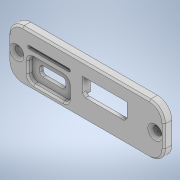
# Autodesk Inventor part: cover
Saved by Autodesk Inventor 2021 (Build 250183000, 183)
## iProperties
Created: 2025-12-12
Part Number: cover
Material: Generic
Document SubType Name: Modeling
Designer: Toby
Density: 1 g/cm^3
Appearance: Default
Author: Toby
Autodesk Inventor part; units mm, degrees
ref_plane "YZ Plane" through (0, 0, 0) normal (1, 0, 0) x (0, 1, 0)
ref_plane "XZ Plane" through (0, 0, 0) normal (0, 1, 0) x (-1, 0, 0)
ref_plane "XY Plane" through (0, 0, 0) normal (0, 0, 1) x (1, 0, 0)
sketch "Sketch1" plane through (0, 0, 0) normal (0, 0, 1) x (1, 0, 0)
  line L0 (-27, 8.75) -> (27, 8.75)
  line L1 (27, 8.75) -> (27, -8.75)
  line L2 (27, -8.75) -> (-27, -8.75)
  line L3 (-27, -8.75) -> (-27, 8.75)
  point P0 (0, 0)
  dimension "d0" = 17.5
  dimension "d1" = 54
  dimension "d2" = 8.75
  dimension "d3" = 27
  constraints: 8 end point, 2 parallel, 1 horizontal, 1 perpendicular
  measures "d0" distance of L2.end L0.start
  measures "d1" distance of L0.start L0.end
  measures "d2" distance from line of point (0, 0) L0
  measures "d3" distance from line of point (0, 0) L3
extrude "Extrusion1" add sketch "Sketch1" along normal blind 2.8
fillet "Fillet1" radius 5 4 edges at (-27, 8.75, 1.4) (-27, -8.75, 1.4) (27, 8.75, 1.4) (27, -8.75, 1.4)
sketch "Sketch2" plane through (0, 0, 2.8) normal (0, 0, 1) x (1, 0, 0)
  line L0 (-22, -8.75) -> (22, -8.75) projected
  line L1 (-27, 3.75) -> (-27, -3.75) projected
  line L2 (27, -3.75) -> (27, 3.75) projected
  point P0 (0, 0)
  point P1 (-24, 0)
  point P2 (24, 0)
  dimension "d7" = 8.75
  dimension "d8" = 8.75
  dimension "d9" = 3
  dimension "d10" = 3
  measures "d7" distance from line of L0 point (-24, 0)
  measures "d8" distance from line of L0 point (24, 0)
  measures "d9" distance from line of L1 point (-24, 0)
  measures "d10" distance from line of L2 point (24, 0)
hole "Hole1" at (-24, 0, 2.8) at (24, 0, 2.8) direction (0, 0, -1) diameter 3 depth 8.8 tip angle 118 countersink diameter 5 countersink angle 90
chamfer "Chamfer1" distance 0.6 angle 45 8 edges at (0, 8.75, 2.8) (-25.5355, 7.2855, 2.8) (-27, 0, 2.8) (-25.5355, -7.2855, 2.8) (0, -8.75, 2.8) (25.5355, -7.2855, 2.8) (27, 0, 2.8) (25.5355, 7.2855, 2.8)
sketch "Sketch3" plane through (0, 0, 2.8) normal (0, 0, 1) x (1, 0, 0)
  line L0 (-21, 6.75) -> (21, 6.75)
  line L1 (21, 6.75) -> (21, -6.75)
  line L2 (21, -6.75) -> (-21, -6.75)
  line L3 (-21, -6.75) -> (-21, 6.75)
  line L4 (22, 8.75) -> (-22, 8.75) projected
  line L5 (-22, -8.75) -> (22, -8.75) projected
  line L6 (-27, 3.75) -> (-27, -3.75) projected
  line L7 (27, -3.75) -> (27, 3.75) projected
  line L8 (-17.6, -1.05) -> (-8.6, -1.05)
  line L9 (-8.6, -1.05) -> (-8.6, -4.55)
  line L10 (-8.6, -4.55) -> (-17.6, -4.55)
  line L11 (-17.6, -4.55) -> (-17.6, -1.05)
  point P0 (0, 0)
  dimension "d21" = 2
  dimension "d22" = 2
  dimension "d23" = 6
  dimension "d24" = 6
  dimension "d25" = 3.4
  dimension "d26" = 9
  dimension "d27" = 3.5
  dimension "d28" = 2.2
  constraints: 16 end point, 4 parallel, 2 horizontal, 2 perpendicular
  measures "d21" distance between parallel lines of L4 L0
  measures "d22" distance between parallel lines of L5 L2
  measures "d23" distance between parallel lines of L6 L3
  measures "d24" distance between parallel lines of L7 L1
  measures "d25" distance between parallel lines of L3 L11
  measures "d26" distance of L8.start L8.end
  measures "d27" distance between parallel lines of L10 L8
  measures "d28" distance between parallel lines of L2 L10
extrude "Extrusion2" cut sketch "Sketch3" against normal blind 2.8 contours L8 L9 L10 L11
sketch "Sketch4" plane through (0, 0, 2.8) normal (0, 0, 1) x (1, 0, 0)
  line L0 (-1.2, 4.25) -> (14.3, 4.25)
  line L1 (14.3, 4.25) -> (14.3, -1.75)
  line L2 (14.3, -1.75) -> (-1.2, -1.75)
  line L3 (-1.2, -1.75) -> (-1.2, 4.25)
  line L4 (22, 8.75) -> (-22, 8.75) projected
  line L5 (-27, 3.75) -> (-27, -3.75) projected
  line L6 (-8.6, -4.55) -> (-17.6, -4.55) projected
  point P0 (0, 0)
  dimension "d31" = 15.5
  dimension "d32" = 6
  dimension "d34" = 25.8
  dimension "d35" = 4.5
  dimension "d36" = 2.8
  constraints: 8 end point, 2 parallel, 1 horizontal, 1 perpendicular
  measures "d31" distance of L0.start L0.end
  measures "d32" distance of L2.end L0.start
  measures "d34" distance between parallel lines of L5 L3
  measures "d35" distance between parallel lines of L4 L0
  measures "d36" distance between parallel lines of L2 L6
extrude "Extrusion3" cut sketch "Sketch4" against normal blind 2.8
fillet "Fillet3" radius 1 4 edges at (-8.6, -1.05, 1.4) (-17.6, -1.05, 1.4) (-17.6, -4.55, 1.4) (-8.6, -4.55, 1.4)
chamfer "Chamfer6" distance 0.6 angle 45 8 edges at (-13.1, -1.05, 2.8) (-8.8929, -1.3429, 2.8) (-8.6, -2.8, 2.8) (-8.8929, -4.2571, 2.8) (-13.1, -4.55, 2.8) (-17.3071, -4.2571, 2.8) (-17.6, -2.8, 2.8) (-17.3071, -1.3429, 2.8)
sketch "Sketch7" plane through (0, 0, 2.8) normal (0, 0, 1) x (1, 0, 0)
  line L0 (22, 8.75) -> (-22, 8.75) projected
  line L1 (-22, -8.75) -> (22, -8.75) projected
  line L2 (-20.2, 8.75) -> (-6, 8.75)
  line L3 (-6, 8.75) -> (-6, -8.75)
  line L4 (-6, -8.75) -> (-20.2, -8.75)
  line L5 (-20.2, -8.75) -> (-20.2, 8.75)
  line L6 (-27, 3.75) -> (-27, -3.75) projected
  line L7 (-18.2, -2.05) -> (-18.2, -3.55) projected
  line L8 (-8, -3.55) -> (-8, -2.05) projected
  line L9 (-6, -6.75) -> (-20.2, -6.75)
  line L10 (-20.2, -6.75) -> (-20.2, 1.15)
  line L11 (-20.2, 1.15) -> (-6, 1.15)
  line L12 (-6, 1.15) -> (-6, -6.75)
  line L13 (-9.6, -4.55) -> (-16.6, -4.55) projected
  line L14 (-16.6, -1.05) -> (-9.6, -1.05) projected
  point P0 (0, 0)
  dimension "d66" = 6.8
  dimension "d67" = 21
  dimension "d68" = 2
  dimension "d69" = 2
  dimension "d94" = 2
  dimension "d95" = 7.6
  dimension "d96" = 2.2
  dimension "d97" = 2.2
  constraints: 16 end point, 4 parallel, 4 point on line, 2 horizontal, 2 perpendicular
  measures "d66" distance between parallel lines of L6 L5
  measures "d67" distance between parallel lines of L6 L3
  measures "d68" distance between parallel lines of L7 L5
  measures "d69" distance between parallel lines of L3 L8
  measures "d94" distance between parallel lines of L9 L4
  measures "d95" distance between parallel lines of L2 L11
  measures "d96" distance between parallel lines of L13 L9
  measures "d97" distance between parallel lines of L11 L14
extrude "Extrusion6" cut sketch "Sketch7" against normal blind 1.6 contours L3 L9 L5 L11
chamfer "Chamfer9" distance 1 angle 45 2 edges at (-1.2, -1.75, 1.4) (14.3, -1.75, 1.4)
sketch "Sketch8" plane through (0, 0, 0) normal (0, 0, -1) x (-1, 0, 0)
  line L0 (-18, 4.25) -> (5, 4.25)
  line L1 (5, 4.25) -> (5, -3.75)
  line L2 (5, -3.75) -> (-18, -3.75)
  line L3 (-18, -3.75) -> (-18, 4.25)
  line L4 (-27, -3.75) -> (-27, 3.75) projected
  line L5 (-14.3, 4.25) -> (1.2, 4.25) projected
  line L6 (22, -8.75) -> (-22, -8.75) projected
  line L7 (-14.3, -0.75) -> (-14.3, 4.25) projected
  line L8 (-14.3, 4.25) -> (-18, 4.25)
  line L9 (-18, 4.25) -> (-18, -1.75)
  line L10 (-18, -1.75) -> (-14.3, -1.75)
  line L11 (-14.3, -1.75) -> (-14.3, 4.25)
  line L12 (1.2, 4.25) -> (1.2, -0.75) projected
  line L13 (1.2, 4.25) -> (5, 4.25)
  line L14 (5, 4.25) -> (5, -1.75)
  line L15 (5, -1.75) -> (1.2, -1.75)
  line L16 (1.2, -1.75) -> (1.2, 4.25)
  point P0 (0, 0)
  point P1 (1.2, -0.75)
  dimension "d81" = 9
  dimension "d82" = 32
  dimension "d83" = 5
  dimension "d89" = 2
  dimension "d90" = 2
  constraints: 24 end point, 6 parallel, 3 horizontal, 3 perpendicular, 2 point on line, 1 collinear
  measures "d81" distance between parallel lines of L4 L3
  measures "d82" distance between parallel lines of L4 L1
  measures "d83" distance between parallel lines of L6 L2
  measures "d89" distance between parallel lines of L2 L10
  measures "d90" distance between parallel lines of L2 L15
extrude "Extrusion7" cut sketch "Sketch8" against normal blind 1.6 contours L0 L12 L16 L15 L1 L2 L3 L10 L11 L7
chamfer "Chamfer11" distance 1.6 angle 45 1 edges at (6.5, -3.75, 0)
fillet "Fillet5" radius 2 4 edges at (-20.2, 1.15, 2) (-6, 1.15, 2) (-6, -6.75, 2) (-20.2, -6.75, 2)
chamfer "Chamfer12" distance 0.6 angle 45 8 edges at (-13.1, 1.15, 2.8) (-6.5858, 0.5642, 2.8) (-6, -2.8, 2.8) (-6.5858, -6.1642, 2.8) (-13.1, -6.75, 2.8) (-19.6142, -6.1642, 2.8) (-20.2, -2.8, 2.8) (-19.6142, 0.5642, 2.8)
sketch "Sketch9" plane through (0, 0, 2.8) normal (0, 0, 1) x (1, 0, 0)
  line L0 (-20.2, 4.25) -> (-5.4, 4.25)
  line L1 (-5.4, 4.25) -> (-5.4, 3.25)
  line L2 (-5.4, 3.25) -> (-20.2, 3.25)
  line L3 (-20.2, 3.25) -> (-20.2, 4.25)
  line L4 (-1.2, 4.25) -> (14.3, 4.25) projected
  line L5 (-17.6, -2.05) -> (-17.6, -3.55) projected
  line L6 (-8.6, -3.55) -> (-8.6, -2.05) projected
  line L7 (-20.2, -4.75) -> (-20.2, -0.85) projected
  line L8 (-5.4, -4.75) -> (-5.4, -0.85) projected
  point P0 (0, 0)
  dimension "d102" = 1
  constraints: 8 end point, 3 collinear, 2 parallel, 1 horizontal, 1 perpendicular
  measures "d102" distance between parallel lines of L0 L2
extrude "Extrusion8" cut sketch "Sketch9" against normal blind 3
fillet "Fillet6" radius 0.5 4 edges at (-5.4, 4.25, 1.4) (-5.4, 3.25, 1.4) (-20.2, 3.25, 1.4) (-20.2, 4.25, 1.4)
body "Solid1"
